Benzomatic Oxy-Mapp Torch Oxygen Regulator Knob (Autodesk Fusion 360 design; units mm, degrees)
Autodesk Fusion 360 part; units mm, degrees
sketch "Sketch1" plane through (0, 0, 0) normal (0, 0, 1) x (1, 0, 0)
  circle A0 centre (0, 0) radius 15
  dimension "d1" = 30
  constraint coincident A0.centre origin
  measures "d1" diameter of A0
extrude "Extrude1" add sketch "Sketch1" along normal blind 14
sketch "Sketch2" plane through (0, 0, 0) normal (0, 0, -1) x (1, 0, 0)
  circle A0 centre (0, 0) radius 15
  circle A1 centre (0, 0) radius 6.25
  dimension "d4" = 12.5
  constraint coincident A0.centre A1.centre
  measures "d4" diameter of A1
extrude "Extrude2" cut sketch "Sketch2" against normal blind 9 contours A1
fillet "Fillet1" radius 1.4224 1 edges at (-13.9849, -5.4242, 14)
sketch "Sketch3" plane through (0, 0, 14) normal (0, 0, 1) x (-1, 0, 0)
  circle A0 centre (0, 0) radius 13.5776
  circle A1 centre (0, 0) radius 5.4838
  line L0 (8.1096, -4.2311) -> (-8.2475, -4.2311) construction
  line L1 (-8.2475, -4.2311) -> (-8.2475, -7.4061) construction
  line L2 (-8.2475, -7.4061) -> (8.1096, -7.4061) construction
  line L3 (8.1096, -7.4061) -> (8.1096, -4.2311) construction
  text T0 "< On - Off >" font "Arial" height 3.175 align ink ink in box 0 x 0 at (8.1096, -4.2311) x (-1, 0) y (0, -1) spacing 1 kerned height is em
  constraint concentric A0 A1
  constraint perpendicular L0 L1
  constraint parallel L0 L2
  constraint parallel L1 L3
extrude "Extrude3" cut sketch "Sketch3" against normal blind 0.9906 text T0
named bodies: "Torch Knob"
